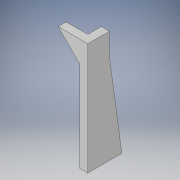
# Autodesk Inventor part: WheelIntakeBrace
Saved by Autodesk Inventor 2017 (Build 210142000, 142)
## iProperties
Created: 2017-12-16
Part Number: WheelIntakeBrace
Material: Generic
Document SubType Name: Modeling
Designer: User
Density: 1 g/cm^3
Appearance: Default
Author: User
Autodesk Inventor part; units mm, degrees
ref_plane "YZ Plane" through (0, 0, 0) normal (1, 0, 0) x (0, 1, 0)
ref_plane "XZ Plane" through (0, 0, 0) normal (0, 1, 0) x (-1, 0, 0)
ref_plane "XY Plane" through (0, 0, 0) normal (0, 0, 1) x (1, 0, 0)
sketch "Sketch1" plane through (0, 0, 0) normal (1, 0, 0) x (0, 1, 0)
  line L0 (0, 0) -> (66.04, 0)
  line L1 (66.04, 0) -> (66.04, -12.7)
  line L2 (66.04, -12.7) -> (53.34, -12.7)
  line L3 (0, -12.7) -> (0, 0)
  line L4 (0, 0) -> (0, -20.066)
  line L5 (66.04, -12.7) -> (53.34, -12.7)
  line L6 (53.34, -12.7) -> (0, -20.066)
  dimension "d0" = 66.04
  dimension "d1" = 12.7
  dimension "d2" = 20.066
  dimension "d3" = 12.7
  constraints: 14 end point, 2 parallel, 1 horizontal, 1 perpendicular, 1 point on line
  measures "d0" distance of L1.end L3.start
  measures "d1" distance of L0.end L1.end
  measures "d2" distance of L0.start L4.end
  measures "d3" distance of L2.end L1.end
extrude "Extrusion1" add sketch "Sketch1" along normal blind 4.7625
sketch "Sketch2" plane through (0, 0, 0) normal (0, 0, 1) x (1, 0, 0)
  line L0 (0, 66.04) -> (4.7625, 66.04) projected
  line L1 (0, 66.04) -> (-12.7, 66.04)
  line L2 (0, 53.34) -> (0, 66.04) projected
  line L3 (-12.7, 66.04) -> (0, 53.34)
  line L4 (0, 53.34) -> (0, 66.04)
  point P0 (0, 0)
  dimension "d6" = 12.7
  constraints: 6 end point, 1 horizontal, 1 perpendicular
  measures "d6" distance of L0.start L1.end
extrude "Extrusion2" add sketch "Sketch2" against normal blind 4.7625
body "Solid1"
